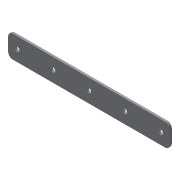
# Autodesk Inventor part: super3
Saved by Autodesk Inventor 2015 SP1 (Build 190203100, 203)
## iProperties
Created: 2015-01-18
Part Number: super3
Material: Generic
Document SubType Name: Sheet Metal
Designer: Owner
Density: 1 g/cm^3
Sheet Metal Rule: Default
Appearance: Default
Author: Owner
Autodesk Inventor part; units mm, degrees
ref_plane "YZ Plane" through (0, 0, 0) normal (1, 0, 0) x (0, 1, 0)
ref_plane "XZ Plane" through (0, 0, 0) normal (0, 1, 0) x (-1, 0, 0)
ref_plane "XY Plane" through (0, 0, 0) normal (0, 0, 1) x (1, 0, 0)
sketch "Sketch1" plane through (0, 0, 0) normal (0, 0, 1) x (1, 0, 0)
  line L0 (0, 0) -> (228.6, 0)
  line L1 (228.6, 0) -> (228.6, 31.75)
  line L2 (228.6, 31.75) -> (0, 31.75)
  line L3 (0, 31.75) -> (0, 0)
  circle A0 centre (215.9, 15.875) radius 3.1623
  line L4 (-50.8, 0) -> (177.8, 0)
  circle A1 centre (165.1, 15.875) radius 3.1623
  line L5 (-101.6, 0) -> (127, 0)
  circle A2 centre (114.3, 15.875) radius 3.1623
  line L6 (-152.4, 0) -> (76.2, 0)
  circle A3 centre (63.5, 15.875) radius 3.1623
  line L7 (-203.2, 0) -> (25.4, 0)
  circle A4 centre (12.7, 15.875) radius 3.1623
  dimension "d0" = 228.6
  dimension "d1" = 31.75
  dimension "d2" = 6.3246
  dimension "d3" = 12.7
  dimension "d4" = 15.875
  dimension "d7" = 50.8
  measures "d0" distance of L2.end L1.end
  measures "d1" distance between parallel lines of L0 L2
  measures "d2" diameter of A0
  measures "d3" distance from line of A0.centre L1
  measures "d4" distance from line of A0.centre L0
  measures "d7" distance of L0.start L4.start
extrude "Plate1" add sketch "Sketch1" along normal blind 3.048
fillet "Corner Round1" radius 6.35 4 edges at (228.6, 31.75, 1.524) (228.6, 0, 1.524) (0, 31.75, 1.524) (0, 0, 1.524)
equation "\"BendRadius\" = Thickness"
equation "\"BendReliefWidth\" = Thickness"
equation "\"BendReliefDepth\" = 0.5 * Thickness"
equation "\"CornerReliefSize\" = 4 * Thickness"
equation "\"MinimumRemnant\" = 2 * Thickness"
equation "\"TransitionRadius\" = BendRadius"
equation "\"JacobiRadiusSize\" = BendRadius"
equation "\"GapSize\" = Thickness"
equation "\"d12\" = BendRadius"
equation "\"Thickness\" = 3.048"
body "Solid1"
